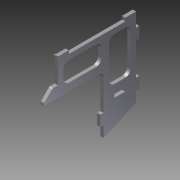
# Autodesk Inventor part: OpenROV 2_2 Ducting Brace
Saved by Autodesk Inventor 2011 (Build 150239000, 239)
## iProperties
Created: 2011-11-04
Part Number: OpenROV 2_2 Ducting Brace
Document SubType Name: Modeling
Designer: user
Density: 1 g/cm^3
Author: user
Autodesk Inventor part; units mm, degrees
ref_plane "YZ Plane" through (0, 0, 0) normal (1, 0, 0) x (0, 1, 0)
ref_plane "XZ Plane" through (0, 0, 0) normal (0, 1, 0) x (-1, 0, 0)
ref_plane "XY Plane" through (0, 0, 0) normal (0, 0, 1) x (1, 0, 0)
sketch "Sketch1" plane through (0, 0, 0) normal (0, 0, 1) x (1, 0, 0)
  point P0 (0, 0)
sketch "Sketch2" plane through (0, 0, 0) normal (1, 0, 0) x (0, 1, 0)
  line L0 (0, 0) -> (-22.95, 0)
  line L1 (-22.95, 0) -> (-22.95, 4.1716)
  line L2 (-23.1803, 0.4176) -> (-23.1803, 0.4176)
  line L3 (-23, -75) -> (-13, -75)
  line L4 (-13, -75) -> (-13, -72)
  line L5 (-13, -72) -> (0, -72)
  line L6 (0, -72) -> (0, -62)
  line L7 (0, -62) -> (-3, -62)
  line L8 (-3, -62) -> (-3, -10)
  line L9 (-3, -10) -> (0, -10)
  line L10 (0, -10) -> (0, 0)
  line L11 (-13, -5) -> (-20.95, -5)
  line L12 (-25.95, -10) -> (-25.95, -35)
  line L13 (-20.95, -40) -> (-13, -40)
  line L14 (-8, -35) -> (-8, -10)
  arc A0 (-8, -10) -> (-13, -5) centre (-13, -10) ccw
  arc A1 (-13, -40) -> (-8, -35) centre (-13, -35) ccw
  arc A2 (-25.95, -35) -> (-20.95, -40) centre (-20.95, -35) ccw
  arc A3 (-20.95, -5) -> (-25.95, -10) centre (-20.95, -10) ccw
  line L15 (-23, -72) -> (-23, -75)
  line L16 (-63, -72) -> (-63, -75)
  line L17 (-63, -75) -> (-53, -75)
  line L18 (-53, -75) -> (-53, -72)
  line L19 (-23, -72) -> (-53, -72)
  line L20 (-63, -72) -> (-73, -72)
  line L21 (-73, -72) -> (-86, -42)
  line L22 (-76, -42) -> (-76, -39)
  line L23 (-76, -39) -> (-66, -39)
  line L24 (-66, -39) -> (-66, -42)
  line L25 (-86, -42) -> (-76, -42)
  line L26 (-66, -42) -> (-37.95, -42)
  line L27 (-13, -47) -> (-43, -47)
  line L28 (-48, -52) -> (-48, -62)
  line L29 (-43, -67) -> (-13, -67)
  line L30 (-8, -62) -> (-8, -52)
  line L31 (-56, -52) -> (-59, -52)
  line L32 (-59, -52) -> (-59, -62)
  line L33 (-59, -62) -> (-56, -62)
  line L34 (-56, -62) -> (-56, -52)
  arc A4 (-8, -52) -> (-13, -47) centre (-13, -52) ccw
  arc A5 (-13, -67) -> (-8, -62) centre (-13, -62) ccw
  arc A6 (-48, -62) -> (-43, -67) centre (-43, -62) ccw
  arc A7 (-43, -47) -> (-48, -52) centre (-43, -52) ccw
  arc A8 (-37.95, -42) -> (-32.95, -37) centre (-37.95, -37) ccw
  line L35 (-32.95, 13) -> (-32.95, -37)
  line L36 (-32.95, 13) -> (-31.7784, 13)
  line L37 (-30.3642, 12.4142) -> (-23.5358, 5.5858)
  arc A9 (-30.3642, 12.4142) -> (-31.7784, 13) centre (-31.7784, 11) ccw
  arc A10 (-22.95, 4.1716) -> (-23.5358, 5.5858) centre (-24.95, 4.1716) ccw
  point P0 (-22.95, 5)
  point P1 (-25.95, -40)
  point P2 (-25.95, -5)
  point P3 (-29.95, -42)
  point P4 (-30.95, 13)
  dimension "d4" = 10
  dimension "d5" = 52
  dimension "d6" = 10
  dimension "d8" = 10
  dimension "d11" = 3
  dimension "d15" = 3
  dimension "d29" = 10
  dimension "d33" = 5
  dimension "d36" = 5
  dimension "d39" = 35
  dimension "d40" = 5
  dimension "d48" = 10
  dimension "d55" = 10
  dimension "d57" = 3
  dimension "d59" = 5
  dimension "d60" = 5
  dimension "d61" = 5
  dimension "d62" = 10
  dimension "d63" = 3
  dimension "d64" = 10
  dimension "d66" = 40
  dimension "d67" = 53
  dimension "d68" = 26.95
  dimension "d69" = 5
  dimension "d75" = 90
  dimension "d76" = 90
  dimension "d77" = 90
  dimension "d78" = 3
  dimension "d79" = 90
  dimension "d80" = 3
  dimension "d81" = 30
  dimension "d82" = 30
  dimension "d83" = 10
  dimension "d84" = 10
  dimension "d85" = 3
  dimension "d86" = 3
  dimension "d87" = 30
  dimension "d89" = 17.95
  dimension "d90" = 5
  dimension "d91" = 13
  dimension "d92" = 32.95
  dimension "d93" = 33.05
  dimension "d94" = 2
  dimension "d95" = 2
  dimension "d96" = 10
  constraints: 76 end point, 22 point on circle, 22 tangent, 17 parallel, 11 centre point, 9 point on line, 8 equal radius, 6 horizontal, 6 perpendicular
  measures "d4" distance of L9.end L0.start
  measures "d5" distance of L7.end L8.end
  measures "d6" distance of L5.end L6.end
  measures "d8" distance of L3.start L3.end
  measures "d11" distance of L8.end L9.end
  measures "d15" distance between parallel lines of L8 L6
  measures "d29" distance between parallel lines of L4 L8
  measures "d33" distance between parallel lines of L0 L11
  measures "d36" distance between parallel lines of L14 L8
  measures "d39" distance of point (-25.95, -5) point (-25.95, -40)
  measures "d40" radius of A0
  measures "d48" distance of L16.end L17.end
  measures "d55" distance of L22.end L23.end
  measures "d57" distance of L23.end L24.end
  measures "d59" distance between parallel lines of L27 L26
  measures "d60" distance between parallel lines of L19 L29
  measures "d61" distance between parallel lines of L8 L30
  measures "d62" distance of L31.end L32.end
  measures "d63" distance of L32.end L33.end
  measures "d64" distance between parallel lines of L26 L31
  measures "d66" distance between parallel lines of L28 L30
  measures "d67" distance between parallel lines of L8 L34
  measures "d68" distance from line of L8 point (-29.95, -42)
  measures "d69" radius of A4
  measures "d75" angle of L19 L18
  measures "d76" angle of L19 L15
  measures "d77" angle of L16 L17
  measures "d78" distance between parallel lines of L19 L3
  measures "d79" angle of L24 L23
  measures "d80" distance of L16.start L16.end
  measures "d81" distance between parallel lines of L26 L19
  measures "d82" distance between parallel lines of L26 L20
  measures "d83" distance from line of L20.end L16
  measures "d84" distance from line of L21.end L22
  measures "d85" distance of L22.start L22.end
  measures "d86" distance of L3.end L4.end
  measures "d87" distance of L15.start L18.end
  measures "d89" distance between parallel lines of L12 L14
  measures "d90" distance of L0.end point (-22.95, 5)
  measures "d91" distance from line of L0 L35.start
  measures "d92" distance between parallel lines of L35 L10
  measures "d93" distance between parallel lines of L24 L35
  measures "d94" distance of L35.start point (-30.95, 13)
  measures "d95" radius of A9
  measures "d96" distance between parallel lines of L35 L1
extrude "Extrusion4" add sketch "Sketch2" along normal blind 3
body "Solid4"
